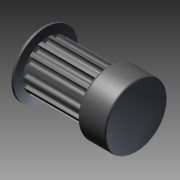
# Autodesk Inventor part: zrr_htd_3m15_0_17031500
Saved by Autodesk Inventor 2011 SP1 (Build 150282100, 282)
## iProperties
Created: 2018-07-07
Part Number: zrr_htd_3m15_0_17031500
Catalog Web Link: www.cadenas.de
Description: zrr_htd_3m15-HTD Pulleys Profile 3M, Timing Belt Width 15mm
Vendor: MAEDLER
Document SubType Name: Modeling
Designer: psAdmin
Manufacturer: MAEDLER
Mass: 11 g
Surface Area: 23.0338 cm^2
Volume: 4.06677 cm^3
Density: 1 g/cm^3
Category: PARTsolutions
Company: MAEDLER
Title: zrr_htd_3m15_0_17031500
Author: Cadenas PARTsolutions
Comments: HTD Pulleys Profile 3M, Timing Belt Width 15mm
PSOL_IDENT_0: {$CADENAS_DATA\23d-libs\maedler\antriebselemente\zahnriemenraeder_zahnriemen\zahnriemenraeder\htd-pr
PSOL_IDENT_1: ofil\zrr_htd_3m15.prj},197 {VTYP=3D},{NB=zrr_htd_3m15_0_17031500},{LINA=zrr_htd_3m15_0_17031500},{NN=
PSOL_IDENT_2: zrr_htd_3m15},{DATE=16.06.2017 10:47:49},{GEOMDATE=09.06.2016 09:07:07},{VERSION=},{LINEID=240},{LIN
PSOL_IDENT_3: ESUBID=-1},{WBVAR=BX}  {NB=zrr_htd_3m15_0_17031500},{LINA=zrr_htd_3m15_0_17031500},{KT=DUMMY},{ARTNR=
PSOL_IDENT_4: 17031500},{PDF=PDF Katalogseite},{AUSF=15-3M-15-0F},{MAT=Aluminium},{ZTL=3.000},{ZRB=15.000},{Z=15.0
PSOL_IDENT_5: 00},{AUS=0F},{ZS=13.560},{BS=18.000},{DO=14.320},{ND=17.500},{B=17.000},{L=26.000},{I=0.000},{VB=0.0
PSOL_IDENT_6: 00},{FB=7.000},{BX=0},{GEW=11.000},{ZT=1.200},{ZB=1.800},{T=0.000},{BB=1.000}
NN: zrr_htd_3m15
NT: HTD-Zahnriemenräder Profil 3M, Zahnriemenbreite 15mm
NB: zrr_htd_3m15_0_17031500
NBSYN: zrr_htd_3m15_$BX._$ARTNR.
LINA: zrr_htd_3m15_0_17031500
ARTNR: 17031500
PDF: PDF Katalogseite
AUSF: 15-3M-15-0F
MAT: Aluminium
ZTL: 3.000
ZRB: 15.000
Z: 15.000
AUS: 0F
ZS: 13.560
BS: 18.000
DO: 14.320
ND: 17.500
B: 17.000
L: 26.000
I: 0.000
VB: 0.000
FB: 7.000
BX: 0
GEW: 11.000
ZT: 1.200
ZB: 1.800
T: 0.000
BB: 1.000
SUPPLIER: MAEDLER
ARTICLENO: zrr_htd_3m15_0_17031500
BOMINFO: zrr_htd_3m15_0_17031500
CREATOR: CADENAS GmbH
Autodesk Inventor part; units mm, degrees
ref_plane "YZ Plane" through (0, 0, 0) normal (1, 0, 0) x (0, 1, 0)
ref_plane "XZ Plane" through (0, 0, 0) normal (0, 1, 0) x (-1, 0, 0)
ref_plane "XY Plane" through (0, 0, 0) normal (0, 0, 1) x (1, 0, 0)
sketch "Sketch_1" plane through (0, 0, 0) normal (0, 0, 1) x (1, 0, 0)
  line L0 (500, 0) -> (-500, 0)
  line L1 (0.3914, 0) -> (0.3914, 6.78)
  line L2 (0.3914, 6.78) -> (0, 9)
  line L3 (0, 9) -> (0.6086, 9)
  line L4 (0.6086, 9) -> (1, 6.78)
  line L5 (1, 6.78) -> (18, 6.78)
  line L6 (18, 6.78) -> (18, 7.75)
  arc A0 (19, 8.75) -> (18, 7.75) centre (19, 7.75) ccw
  line L7 (19, 8.75) -> (25.5, 8.75)
  arc A1 (26, 8.25) -> (25.5, 8.75) centre (25.5, 8.25) ccw
  line L8 (26, 8.25) -> (26, 0)
  line L9 (26, 0) -> (0.3914, 0)
  constraints: 20 end point, 4 point on circle, 2 centre point
revolve "Revolution1" add sketch "Sketch_1" angle 360 about axis through (500, 0, 0) along (1, 0, 0)
sketch "Sketch_2" plane through (1, 0, 0) normal (1, 0, 0) x (0, 0, -1)
  circle A0 centre (0, 0) radius 13.56
  line L0 (-6.7773, 0.1926) -> (-6.5386, 0.2177)
  arc A1 (-5.5494, -0.5833) -> (-6.5386, 0.2177) centre (-6.4445, -0.6773) ccw
  arc A2 (-6.3504, -1.5724) -> (-5.5494, -0.5833) centre (-6.4445, -0.6773) ccw
  line L1 (-6.3504, -1.5724) -> (-6.5891, -1.5975)
  arc A3 (-6.5891, -1.5975) -> (-6.4482, -2.0951) centre (0, 0) ccw
  arc A4 (-6.4482, -2.0951) -> (-6.2697, -2.5806) centre (0, 0) ccw
  line L2 (-6.2697, -2.5806) -> (-6.0618, -2.4606)
  arc A5 (-4.8324, -2.79) -> (-6.0618, -2.4606) centre (-5.6118, -3.24) ccw
  arc A6 (-5.1618, -4.0194) -> (-4.8324, -2.79) centre (-5.6118, -3.24) ccw
  line L3 (-5.1618, -4.0194) -> (-5.3697, -4.1394)
  arc A7 (-5.3697, -4.1394) -> (-5.0385, -4.5367) centre (0, 0) ccw
  arc A8 (-5.0385, -4.5367) -> (-4.678, -4.9076) centre (0, 0) ccw
  line L4 (-4.678, -4.9076) -> (-4.537, -4.7134)
  arc A9 (-3.2798, -4.5143) -> (-4.537, -4.7134) centre (-3.8088, -5.2424) ccw
  arc A10 (-3.0807, -5.7714) -> (-3.2798, -4.5143) centre (-3.8088, -5.2424) ccw
  line L5 (-3.0807, -5.7714) -> (-3.2218, -5.9656)
  arc A11 (-3.2218, -5.9656) -> (-2.7577, -6.1938) centre (0, 0) ccw
  arc A12 (-2.7577, -6.1938) -> (-2.2775, -6.386) centre (0, 0) ccw
  line L6 (-2.2775, -6.386) -> (-2.2276, -6.1513)
  arc A13 (-1.1601, -5.4581) -> (-2.2276, -6.1513) centre (-1.3473, -6.3384) ccw
  arc A14 (-0.4669, -6.5255) -> (-1.1601, -5.4581) centre (-1.3473, -6.3384) ccw
  line L7 (-0.4669, -6.5255) -> (-0.5168, -6.7603)
  arc A15 (-0.5168, -6.7603) -> (0, -6.78) centre (0, 0) ccw
  arc A16 (0, -6.78) -> (0.5168, -6.7603) centre (0, 0) ccw
  line L8 (0.5168, -6.7603) -> (0.4669, -6.5255)
  arc A17 (1.1601, -5.4581) -> (0.4669, -6.5255) centre (1.3473, -6.3384) ccw
  arc A18 (2.2276, -6.1513) -> (1.1601, -5.4581) centre (1.3473, -6.3384) ccw
  line L9 (2.2276, -6.1513) -> (2.2775, -6.386)
  arc A19 (2.2775, -6.386) -> (2.7577, -6.1938) centre (0, 0) ccw
  arc A20 (2.7577, -6.1938) -> (3.2218, -5.9656) centre (0, 0) ccw
  line L10 (3.2218, -5.9656) -> (3.0807, -5.7714)
  arc A21 (3.2798, -4.5143) -> (3.0807, -5.7714) centre (3.8088, -5.2424) ccw
  arc A22 (4.537, -4.7134) -> (3.2798, -4.5143) centre (3.8088, -5.2424) ccw
  line L11 (4.537, -4.7134) -> (4.678, -4.9076)
  arc A23 (4.678, -4.9076) -> (5.0385, -4.5367) centre (0, 0) ccw
  arc A24 (5.0385, -4.5367) -> (5.3697, -4.1394) centre (0, 0) ccw
  line L12 (5.3697, -4.1394) -> (5.1618, -4.0194)
  arc A25 (4.8324, -2.79) -> (5.1618, -4.0194) centre (5.6118, -3.24) ccw
  arc A26 (6.0618, -2.4606) -> (4.8324, -2.79) centre (5.6118, -3.24) ccw
  line L13 (6.0618, -2.4606) -> (6.2697, -2.5806)
  arc A27 (6.2697, -2.5806) -> (6.4482, -2.0951) centre (0, 0) ccw
  arc A28 (6.4482, -2.0951) -> (6.5891, -1.5975) centre (0, 0) ccw
  line L14 (6.5891, -1.5975) -> (6.3504, -1.5724)
  arc A29 (5.5494, -0.5833) -> (6.3504, -1.5724) centre (6.4445, -0.6773) ccw
  arc A30 (6.5386, 0.2177) -> (5.5494, -0.5833) centre (6.4445, -0.6773) ccw
  line L15 (6.5386, 0.2177) -> (6.7773, 0.1926)
  arc A31 (6.7773, 0.1926) -> (6.7429, 0.7087) centre (0, 0) ccw
  arc A32 (6.7429, 0.7087) -> (6.6692, 1.2206) centre (0, 0) ccw
  line L16 (6.6692, 1.2206) -> (6.441, 1.1465)
  arc A33 (5.3069, 1.7243) -> (6.441, 1.1465) centre (6.1628, 2.0024) ccw
  arc A34 (5.8847, 2.8584) -> (5.3069, 1.7243) centre (6.1628, 2.0024) ccw
  line L17 (5.8847, 2.8584) -> (6.113, 2.9325)
  arc A35 (6.113, 2.9325) -> (5.8717, 3.39) centre (0, 0) ccw
  arc A36 (5.8717, 3.39) -> (5.5962, 3.8277) centre (0, 0) ccw
  line L18 (5.5962, 3.8277) -> (5.4178, 3.6671)
  arc A37 (4.1467, 3.7337) -> (5.4178, 3.6671) centre (4.8156, 4.336) ccw
  arc A38 (4.2134, 5.0048) -> (4.1467, 3.7337) centre (4.8156, 4.336) ccw
  line L19 (4.2134, 5.0048) -> (4.3917, 5.1654)
  arc A39 (4.3917, 5.1654) -> (3.9852, 5.4851) centre (0, 0) ccw
  arc A40 (3.9852, 5.4851) -> (3.5555, 5.773) centre (0, 0) ccw
  line L20 (3.5555, 5.773) -> (3.4578, 5.5537)
  arc A41 (2.2696, 5.0976) -> (3.4578, 5.5537) centre (2.6357, 5.9198) ccw
  arc A42 (1.8135, 6.2858) -> (2.2696, 5.0976) centre (2.6357, 5.9198) ccw
  line L21 (1.8135, 6.2858) -> (1.9111, 6.5051)
  arc A43 (1.9111, 6.5051) -> (1.4096, 6.6318) centre (0, 0) ccw
  arc A44 (1.4096, 6.6318) -> (0.9, 6.72) centre (0, 0) ccw
  line L22 (0.9, 6.72) -> (0.9, 6.48)
  arc A45 (0, 5.58) -> (0.9, 6.48) centre (0, 6.48) ccw
  arc A46 (-0.9, 6.48) -> (0, 5.58) centre (0, 6.48) ccw
  line L23 (-0.9, 6.48) -> (-0.9, 6.72)
  arc A47 (-0.9, 6.72) -> (-1.4096, 6.6318) centre (0, 0) ccw
  arc A48 (-1.4096, 6.6318) -> (-1.9111, 6.5051) centre (0, 0) ccw
  line L24 (-1.9111, 6.5051) -> (-1.8135, 6.2858)
  arc A49 (-2.2696, 5.0976) -> (-1.8135, 6.2858) centre (-2.6357, 5.9198) ccw
  arc A50 (-3.4578, 5.5537) -> (-2.2696, 5.0976) centre (-2.6357, 5.9198) ccw
  line L25 (-3.4578, 5.5537) -> (-3.5555, 5.773)
  arc A51 (-3.5555, 5.773) -> (-3.9852, 5.4851) centre (0, 0) ccw
  arc A52 (-3.9852, 5.4851) -> (-4.3917, 5.1654) centre (0, 0) ccw
  line L26 (-4.3917, 5.1654) -> (-4.2134, 5.0048)
  arc A53 (-4.1467, 3.7337) -> (-4.2134, 5.0048) centre (-4.8156, 4.336) ccw
  arc A54 (-5.4178, 3.6671) -> (-4.1467, 3.7337) centre (-4.8156, 4.336) ccw
  line L27 (-5.4178, 3.6671) -> (-5.5962, 3.8277)
  arc A55 (-5.5962, 3.8277) -> (-5.8717, 3.39) centre (0, 0) ccw
  arc A56 (-5.8717, 3.39) -> (-6.113, 2.9325) centre (0, 0) ccw
  line L28 (-6.113, 2.9325) -> (-5.8847, 2.8584)
  arc A57 (-5.3069, 1.7243) -> (-5.8847, 2.8584) centre (-6.1628, 2.0024) ccw
  arc A58 (-6.441, 1.1465) -> (-5.3069, 1.7243) centre (-6.1628, 2.0024) ccw
  line L29 (-6.441, 1.1465) -> (-6.6692, 1.2206)
  arc A59 (-6.6692, 1.2206) -> (-6.7429, 0.7087) centre (0, 0) ccw
  arc A60 (-6.7429, 0.7087) -> (-6.7773, 0.1926) centre (0, 0) ccw
  constraints: 120 point on circle, 61 centre point, 60 end point
extrude "Extrusion1" cut sketch "Sketch_2" along normal blind 17
body "Solid1"
